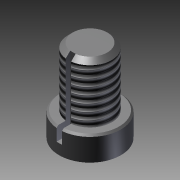
# Autodesk Inventor part: MBS1-bushings
Saved by Autodesk Inventor 2015 (Build 190159000, 159)
## iProperties
Category: PARTsolutions
Company: NKKSWITCHES
Created: 2015-01-04
Part Number: MBS1-bushings
Catalog Web Link: www.cadenas.de
Description: MB2000 Series - Bushing Mount Miniature Pushbuttons -bushings-
Vendor: NKKSWITCHES
Document SubType Name: Modeling
Designer: PARTuser1
Manufacturer: NKKSWITCHES
Mass: 0.479836 g
Surface Area: 4.02457 cm^2
Volume: 0.479836 cm^3
Density: 1 g/cm^3
Material: Generic
Appearance: PSOLRGB-242-242-242
PSOL_IDENT_0: {$CADENAS_DATA\23d-libs\nkkswitches\pushbuttons\mb2000\parts\mb2000_bm_bushings.prj},228 {VTYP=3D},{
PSOL_IDENT_1: NB=MBS1-bushings},{LINA=MBS1-bushings},{NN=MB2000 Series - Bushing Mount Miniature Pushbuttons -bush
PSOL_IDENT_2: ings},{DATE=21.11.2014 08:56:24},{GEOMDATE=19.02.2009 11:25:00},{VERSION=},{LINEID=10},{LINESUBID=-1
PSOL_IDENT_3: },{WBVAR=BSHNG}  {NB=MBS1-bushings},{LINA=MBS1-bushings},{KT=DUMMY},{PN=MBS1},{SRS=MB},{BSHNG=S1},{D=
PSOL_IDENT_4: 0.250},{M=6}
SUPPLIER: NKKSWITCHES
ARTICLENO: MBS1-bushings
BOMINFO: MBS1-bushings
CREATOR: CADENAS GmbH
Title: MBS1-bushings
Author: Cadenas PARTsolutions
Autodesk Inventor part; units mm, degrees
sketch "Sketch_1" plane through (0, 0, 0) normal (1, 0, 0) x (0, 1, 0)
  line L0 (0, 0) -> (12.0142, 0)
  line L1 (12.0142, 0) -> (12.0142, -2.5311)
  line L2 (12.0142, -2.5311) -> (11.3703, -3.175)
  line L3 (11.3703, -3.175) -> (3.5052, -3.175)
  line L4 (3.5052, -3.175) -> (3.5052, -4.2418)
  line L5 (3.5052, -4.2418) -> (3.2512, -4.4958)
  line L6 (3.2512, -4.4958) -> (0, -4.4958)
  line L7 (0, -4.4958) -> (0, 0)
  line L8 (0, 0) -> (12.0142, 0)
  constraints: 18 end point
revolve "Revolution1" add sketch "Sketch_1" angle 360 about axis through (0, 0, 0) along (0, -1, 0)
thread "Thread1" size "1/4-24 UNS" class "2A" standard "ANSI Unified Screw Threads" full length
sketch "Sketch_3" plane through (0, 1.524, 0) normal (0, 1, 0) x (1, 0, 0)
  line L0 (-0.3937, -2.4892) -> (-0.3937, -6.2992)
  line L1 (-0.3937, -6.2992) -> (0.3937, -6.2992)
  line L2 (0.3937, -6.2992) -> (0.3937, -2.4892)
  line L3 (0.3937, -2.4892) -> (-0.3937, -2.4892)
  constraints: 8 end point
extrude "Extrusion1" cut sketch "Sketch_3" along normal blind 12.192
ref_plane "at507_XY" through (0, 5.3975, 0) normal (0, -1, 0) x (1, 0, 0)
ref_plane "at507_YZ" through (0, 5.3975, 0) normal (1, 0, 0) x (0, 0, 1)
ref_plane "at507_ZX" through (0, 5.3975, 0) normal (0, 0, 1) x (0, -1, 0)
ref_plane "at513_XY" through (0, 3.5052, 0) normal (0, 1, 0) x (1, 0, 0)
ref_plane "at513_YZ" through (0, 3.5052, 0) normal (1, 0, 0) x (0, 0, -1)
ref_plane "at513_ZX" through (0, 3.5052, 0) normal (0, 0, -1) x (0, 1, 0)
ref_plane "at516_XY" through (0, 5.7912, 0) normal (0, 1, 0) x (1, 0, 0)
ref_plane "at516_YZ" through (0, 5.7912, 0) normal (1, 0, 0) x (0, 0, -1)
ref_plane "at516_ZX" through (0, 5.7912, 0) normal (0, 0, -1) x (0, 1, 0)
ref_plane "to_at509_XY" through (0, 5.7785, 0) normal (0, 1, 0) x (1, 0, 0)
ref_plane "to_at509_YZ" through (0, 5.7785, 0) normal (1, 0, 0) x (0, 0, -1)
ref_plane "to_at509_ZX" through (0, 5.7785, 0) normal (0, 0, -1) x (0, 1, 0)
ref_plane "to_at513_1_XY" through (0, 6.2865, 0) normal (0, 1, 0) x (1, 0, 0)
ref_plane "to_at513_1_YZ" through (0, 6.2865, 0) normal (1, 0, 0) x (0, 0, -1)
ref_plane "to_at513_1_ZX" through (0, 6.2865, 0) normal (0, 0, -1) x (0, 1, 0)
ref_plane "to_bodycover_XY" through (0, 0, 0) normal (0, 1, 0) x (1, 0, 0)
ref_plane "to_bodycover_YZ" through (0, 0, 0) normal (1, 0, 0) x (0, 0, -1)
ref_plane "to_bodycover_ZX" through (0, 0, 0) normal (0, 0, -1) x (0, 1, 0)
ref_plane "to_plunger_XY" through (0, 12.0142, 0) normal (0, -1, 0) x (1, 0, 0)
ref_plane "to_plunger_YZ" through (0, 12.0142, 0) normal (1, 0, 0) x (0, 0, 1)
ref_plane "to_plunger_ZX" through (0, 12.0142, 0) normal (0, 0, 1) x (0, -1, 0)
body "Solid1"
